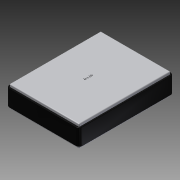
# Autodesk Inventor part: Control System_RadioRobot_DLink_DAP1522
Saved by Autodesk Inventor 2014 SP1 (Build 180222100, 222)
## iProperties
Category: Control System
Company: Autodesk Inc.
Created: 2012-12-01
Part Number: Control System_RadioRobot_DLink_DAP1522
Document SubType Name: Modeling
Designer: Autodesk Inc.
Density: 0.312319 g/cm^3
Catalog Web Link: ftp://ftp10.dlink.com/pdfs/products/DAP-1522/DAP-1522_ds.pdf
Description: Wireless bridge
Vendor: D-Link
Mass: 117.934 g
Surface Area: 482.928 cm^2
Volume: 523.554 cm^3
Material: Generic
Appearance: Glossy - Black
Author: Autodesk Inc.
Autodesk Inventor part; units mm, degrees
note: some values were not read from the file. Chosen so that the rebuilt part matches the saved one: direction of "Emboss1".
ref_plane "YZ Plane" through (0, 0, 0) normal (1, 0, 0) x (0, 1, 0)
ref_plane "XZ Plane" through (0, 0, 0) normal (0, 1, 0) x (-1, 0, 0)
ref_plane "XY Plane" through (0, 0, 0) normal (0, 0, 1) x (1, 0, 0)
sketch "Sketch1" plane through (0, 0, 0) normal (0, 0, 1) x (1, 0, 0)
  line L0 (0, 0) -> (144.78, 0)
  line L1 (144.78, 0) -> (144.78, -111.76)
  line L2 (144.78, -111.76) -> (0, -111.76)
  line L3 (0, -111.76) -> (0, 0)
  dimension "d0" = 144.78
  dimension "d1" = 111.76
  constraints: 8 end point, 2 parallel, 1 horizontal, 1 perpendicular
  measures "d0" distance of L1.end L2.end
  measures "d1" distance of L0.end L1.end
extrude "Extrusion1" add sketch "Sketch1" along normal mid plane 25.4
sketch "Sketch2" plane through (0, 0, 0) normal (0, 0, 1) x (1, 0, 0)
  line L0 (2.54, -109.22) -> (142.24, -109.22)
  line L1 (142.24, -109.22) -> (142.24, -2.54)
  line L2 (142.24, -2.54) -> (2.54, -2.54)
  line L3 (2.54, -2.54) -> (2.54, -109.22)
  line L4 (0, 0) -> (0, -111.76) projected
  line L5 (144.78, 0) -> (0, 0) projected
  dimension "d4" = 2.54
  dimension "d5" = 2.54
  dimension "d11" = 2.54
  dimension "d12" = 2.54
  constraints: 8 end point, 2 parallel, 1 horizontal, 1 perpendicular
  measures "d4" distance between parallel lines of L3 L4
  measures "d5" distance between parallel lines of L5 L2
  measures "d11" distance from line of L4.end L0
  measures "d12" distance from line of L5.start L1
extrude "Extrusion2" add sketch "Sketch2" along normal mid plane 33.02
fillet "Fillet1" radius 0.508 8 edges at (0, -55.88, 12.7) (72.39, -111.76, 12.7) (144.78, -55.88, 12.7) (72.39, 0, 12.7) (0, -55.88, -12.7) (72.39, 0, -12.7) (72.39, -111.76, -12.7) (144.78, -55.88, -12.7)
fillet "Fillet2" radius 1.27 16 edges at (2.54, -55.88, 16.51) (72.39, -2.54, 16.51) (142.24, -55.88, 16.51) (72.39, -109.22, 16.51) (2.54, -109.22, 14.605) (142.24, -109.22, 14.605) (142.24, -2.54, 14.605) (2.54, -2.54, 14.605) (2.54, -55.88, -16.51) (72.39, -109.22, -16.51) (142.24, -55.88, -16.51) (72.39, -2.54, -16.51) (142.24, -2.54, -14.605) (2.54, -2.54, -14.605) (2.54, -109.22, -14.605) (142.24, -109.22, -14.605)
fillet "Fillet3" radius 5.08 12 edges at (0.1488, -0.1488, 12.5512) (0.1488, -0.1488, -12.5512) (0, 0, 0) (0.1488, -111.6112, -12.5512) (0.1488, -111.6112, 12.5512) (0, -111.76, 0) (144.6312, -111.6112, -12.5512) (144.6312, -111.6112, 12.5512) (144.78, -111.76, 0) (144.6312, -0.1488, -12.5512) (144.6312, -0.1488, 12.5512) (144.78, 0, 0)
sketch "Sketch3" plane through (0, 0, 16.51) normal (0, 0, 1) x (1, 0, 0)
  line L0 (65.3497, -52.5642) -> (65.3318, -52.6773)
  line L1 (66.6099, -52.5642) -> (65.3497, -52.5642)
  spline S0 degree 3 poles (67.8153, -52.9891) (67.5735, -52.7056) (67.1714, -52.5642) (66.6099, -52.5642) knots 0 0 0 0 1 1 1 1
  ellipse E0 centre (41.2685, -67.4041) end of major axis (67.9555, -53.1944) minor radius 5.823 (68.0717, -54.0812) -> (67.8153, -52.9891) ccw
  ellipse E1 centre (-43.6594, 9.5813) end of major axis (67.8598, -54.6923) minor radius 14.6191 (67.4733, -55.152) -> (68.0717, -54.0812) ccw
  spline S1 degree 3 poles (66.1223, -55.5743) (66.6925, -55.5743) (67.1412, -55.435) (67.4733, -55.152) knots 0 0 0 0 1 1 1 1
  line L2 (64.873, -55.5743) -> (66.1223, -55.5743)
  line L3 (64.8909, -55.4611) -> (64.873, -55.5743)
  spline S2 degree 3 poles (65.2131, -55.368) (65.1492, -55.4241) (65.0421, -55.4545) (64.8909, -55.4611) knots 0 0 0 0 1 1 1 1
  ellipse E2 centre (64.1895, -52.8955) end of major axis (63.2262, -50.386) minor radius 0.7127 (65.2131, -55.368) -> (65.3425, -55.0693) ccw
  line L4 (65.3425, -55.0693) -> (65.6445, -53.1627)
  spline S3 degree 3 poles (65.6237, -52.7579) (65.6728, -52.8057) (65.6797, -52.9407) (65.6445, -53.1627) knots 0 0 0 0 1 1 1 1
  spline S4 degree 3 poles (65.3318, -52.6773) (65.4766, -52.6839) (65.5747, -52.71) (65.6237, -52.7579) knots 0 0 0 0 1 1 1 1
  line L5 (68.3955, -54.3728) -> (68.3503, -54.6579)
  line L6 (69.5273, -54.3728) -> (68.3955, -54.3728)
  line L7 (69.4821, -54.6579) -> (69.5273, -54.3728)
  line L8 (68.3503, -54.6579) -> (69.4821, -54.6579)
  line L9 (69.6596, -55.4611) -> (69.6417, -55.5743)
  ellipse E3 centre (57.3747, -50.2312) end of major axis (70.0338, -55.3094) minor radius 1.3637 (69.6596, -55.4611) -> (70.0293, -55.3193) ccw
  spline S5 degree 3 poles (70.1261, -54.9757) (70.1158, -55.0406) (70.1023, -55.1074) (70.0705, -55.2204) (70.0523, -55.2729) (70.0293, -55.3193) knots 0 0 0 0 0.558026 0.558026 1 1 1 1
  line L10 (70.4132, -53.1627) -> (70.1261, -54.9757)
  spline S6 degree 3 poles (70.4099, -52.7992) (70.4261, -52.8431) (70.4315, -52.8969) (70.4326, -53.0177) (70.4241, -53.0937) (70.4132, -53.1627) knots 0 0 0 0 0.421499 0.421499 1 1 1 1
  spline S7 degree 3 poles (70.1005, -52.6773) (70.2776, -52.686) (70.3824, -52.7252) (70.4099, -52.7992) knots 0 0 0 0 1 1 1 1
  line L11 (70.1184, -52.5642) -> (70.1005, -52.6773)
  line L12 (71.3677, -52.5642) -> (70.1184, -52.5642)
  line L13 (71.3498, -52.6773) -> (71.3677, -52.5642)
  spline S8 degree 3 poles (70.9984, -52.7796) (71.0444, -52.723) (71.1606, -52.6904) (71.3498, -52.6773) knots 0 0 0 0 1 1 1 1
  spline S9 degree 3 poles (70.8833, -53.1627) (70.9151, -52.9625) (70.9525, -52.8362) (70.9984, -52.7796) knots 0 0 0 0 1 1 1 1
  line L14 (70.5786, -55.0867) -> (70.8833, -53.1627)
  spline S10 degree 3 poles (70.6211, -55.3396) (70.5689, -55.3131) (70.5562, -55.2282) (70.5786, -55.0867) knots 0 0 0 0 1 1 1 1
  ellipse E4 centre (77.9872, -54.0432) end of major axis (85.3798, -52.7746) minor radius 0.4222 (70.6211, -55.3396) -> (70.9851, -55.3784) ccw
  line L15 (71.1788, -55.3784) -> (70.9851, -55.3784)
  spline S11 degree 3 poles (71.7877, -55.2717) (71.6284, -55.3435) (71.4248, -55.3784) (71.1788, -55.3784) knots 0 0 0 0 1 1 1 1
  ellipse E5 centre (72.6832, 50.9705) end of major axis (73.757, 157.2522) minor radius 6.3937 (71.7877, -55.2717) -> (72.2664, -54.7646) ccw
  line L16 (72.3774, -54.7646) -> (72.2664, -54.7646)
  line L17 (72.0206, -55.5743) -> (72.3774, -54.7646)
  line L18 (69.6417, -55.5743) -> (72.0206, -55.5743)
  line L19 (72.4733, -55.5743) -> (73.481, -55.5743)
  line L20 (72.4871, -55.4872) -> (72.4733, -55.5743)
  spline S12 degree 3 poles (72.7487, -55.4023) (72.7005, -55.4589) (72.6133, -55.4872) (72.4871, -55.4872) knots 0 0 0 0 1 1 1 1
  spline S13 degree 3 poles (72.8627, -55.0671) (72.8519, -55.135) (72.8366, -55.2089) (72.7998, -55.3171) (72.7783, -55.3675) (72.7487, -55.4023) knots 0 0 0 0 0.60012 0.60012 1 1 1 1
  line L21 (72.8627, -55.0671) -> (73.0271, -54.0289)
  ellipse E6 centre (72.1534, -55.2391) end of major axis (72.9896, -53.7975) minor radius 0.3276 (73.0271, -54.0289) -> (73.0102, -53.8161) ccw
  spline S14 degree 3 poles (72.841, -53.7612) (72.8757, -53.7612) (72.9141, -53.7643) (72.9602, -53.7793) (72.973, -53.7849) (72.9943, -53.7988) (73.0031, -53.8067) (73.0102, -53.8161) knots 0 0 0 0 0.576408 0.576408 0.803632 0.803632 1 1 1 1
  line L22 (72.7605, -53.7612) -> (72.841, -53.7612)
  line L23 (72.7742, -53.6742) -> (72.7605, -53.7612)
  line L24 (73.507, -53.4587) -> (72.7742, -53.6742)
  line L25 (73.2523, -55.0671) -> (73.507, -53.4587)
  spline S15 degree 3 poles (73.2661, -55.4159) (73.2265, -55.3675) (73.2233, -55.25) (73.2523, -55.0671) knots 0 0 0 0 1 1 1 1
  ellipse E7 centre (77.3295, -52.9371) end of major axis (81.4031, -50.4727) minor radius 0.7662 (73.2661, -55.4159) -> (73.4948, -55.4872) ccw
  line L26 (73.481, -55.5743) -> (73.4948, -55.4872)
  spline S16 degree 3 poles (73.146, -52.7013) (73.1353, -52.7687) (73.1481, -52.8253) (73.1881, -52.8716) knots 0 0 0 0 1 1 1 1
  spline S17 degree 3 poles (73.2425, -52.5315) (73.1871, -52.5794) (73.1563, -52.636) (73.146, -52.7013) knots 0 0 0 0 1 1 1 1
  spline S18 degree 3 poles (73.4258, -52.4597) (73.3584, -52.4597) (73.298, -52.4836) (73.2425, -52.5315) knots 0 0 0 0 1 1 1 1
  spline S19 degree 3 poles (73.5821, -52.5315) (73.5418, -52.4836) (73.4911, -52.4597) (73.4258, -52.4597) knots 0 0 0 0 1 1 1 1
  spline S20 degree 3 poles (73.627, -52.7013) (73.6373, -52.636) (73.6224, -52.5794) (73.5821, -52.5315) knots 0 0 0 0 1 1 1 1
  ellipse E8 centre (71.9698, -51.7105) end of major axis (73.582, -52.8173) minor radius 0.7104 (73.5276, -52.8754) -> (73.627, -52.7013) ccw
  spline S21 degree 3 poles (73.3497, -52.9407) (73.415, -52.9407) (73.4728, -52.9189) (73.5276, -52.8754) knots 0 0 0 0 1 1 1 1
  spline S22 degree 3 poles (73.1881, -52.8716) (73.229, -52.9189) (73.2822, -52.9407) (73.3497, -52.9407) knots 0 0 0 0 1 1 1 1
  line L27 (73.6167, -55.4872) -> (73.6029, -55.5743)
  spline S23 degree 3 poles (73.8749, -55.3852) (73.8199, -55.4545) (73.7342, -55.4872) (73.6167, -55.4872) knots 0 0 0 0 1 1 1 1
  spline S24 degree 3 poles (73.9923, -55.0671) (73.9824, -55.1294) (73.9678, -55.1936) (73.9288, -55.2992) (73.9058, -55.3464) (73.8749, -55.3852) knots 0 0 0 0 0.558687 0.558687 1 1 1 1
  line L28 (73.9923, -55.0671) -> (74.1609, -54.0028)
  spline S25 degree 3 poles (74.1506, -53.82) (74.1706, -53.8592) (74.174, -53.9201) (74.1609, -54.0028) knots 0 0 0 0 1 1 1 1
  spline S26 degree 3 poles (74.0163, -53.7612) (74.0859, -53.7612) (74.1307, -53.7808) (74.1506, -53.82) knots 0 0 0 0 1 1 1 1
  line L29 (73.8901, -53.7612) -> (74.0163, -53.7612)
  line L30 (73.9038, -53.6742) -> (73.8901, -53.7612)
  line L31 (74.6366, -53.4587) -> (73.9038, -53.6742)
  line L32 (74.5839, -53.7917) -> (74.6366, -53.4587)
  spline S27 degree 3 poles (74.9832, -53.524) (74.8806, -53.5675) (74.7489, -53.6568) (74.5839, -53.7917) knots 0 0 0 0 1 1 1 1
  spline S28 degree 3 poles (75.2918, -53.4587) (75.1873, -53.4587) (75.0859, -53.4805) (74.9832, -53.524) knots 0 0 0 0 1 1 1 1
  ellipse E9 centre (69.491, -60.1714) end of major axis (63.3694, -66.779) minor radius 1.7408 (75.6688, -53.6311) -> (75.2918, -53.4587) ccw
  ellipse E10 centre (64.3467, -63.1911) end of major axis (75.6367, -53.5878) minor radius 2.4275 (75.7313, -54.1051) -> (75.6688, -53.6311) ccw
  line L33 (75.7313, -54.1051) -> (75.579, -55.0671)
  ellipse E11 centre (79.0817, -48.7921) end of major axis (82.5408, -42.1531) minor radius 0.7356 (75.579, -55.0671) -> (75.6022, -55.4154) ccw
  spline S29 degree 3 poles (75.8215, -55.4872) (75.7192, -55.4872) (75.6468, -55.4633) (75.6022, -55.4154) knots 0 0 0 0 1 1 1 1
  line L34 (75.8077, -55.5743) -> (75.8215, -55.4872)
  line L35 (74.8, -55.5743) -> (75.8077, -55.5743)
  line L36 (74.8138, -55.4872) -> (74.8, -55.5743)
  spline S30 degree 3 poles (75.0576, -55.4148) (74.9982, -55.4633) (74.9182, -55.4872) (74.8138, -55.4872) knots 0 0 0 0 1 1 1 1
  ellipse E12 centre (74.402, -53.5777) end of major axis (73.7975, -51.7123) minor radius 0.5398 (75.0576, -55.4148) -> (75.178, -55.139) ccw
  line L37 (75.178, -55.139) -> (75.3266, -54.2009)
  ellipse E13 centre (55.6406, -76.8384) end of major axis (75.2465, -53.7648) minor radius 2.5286 (75.3266, -54.2009) -> (75.0609, -53.7068) ccw
  ellipse E14 centre (70.9828, -106.1576) end of major axis (75.0958, -53.7082) minor radius 4.8337 (75.0609, -53.7068) -> (74.6474, -53.8853) ccw
  line L38 (74.5573, -53.9593) -> (74.6474, -53.8853)
  line L39 (74.3819, -55.0671) -> (74.5573, -53.9593)
  spline S31 degree 3 poles (74.4075, -55.4001) (74.3639, -55.3457) (74.3553, -55.2347) (74.3819, -55.0671) knots 0 0 0 0 1 1 1 1
  ellipse E15 centre (77.9499, -52.5696) end of major axis (81.4925, -49.7392) minor radius 0.9098 (74.4075, -55.4001) -> (74.6244, -55.4872) ccw
  line L40 (74.6106, -55.5743) -> (74.6244, -55.4872)
  line L41 (73.6029, -55.5743) -> (74.6106, -55.5743)
  line L42 (75.8607, -55.4872) -> (75.8469, -55.5743)
  spline S32 degree 3 poles (76.1147, -55.4088) (76.0636, -55.4567) (75.9789, -55.4828) (75.8607, -55.4872) knots 0 0 0 0 1 1 1 1
  spline S33 degree 3 poles (76.2194, -55.1738) (76.2119, -55.2209) (76.1998, -55.2692) (76.1644, -55.3485) (76.1432, -55.3822) (76.1147, -55.4088) knots 0 0 0 0 0.549628 0.549628 1 1 1 1
  line L43 (76.2194, -55.1738) -> (76.5386, -53.1583)
  spline S34 degree 3 poles (76.5308, -52.8776) (76.5577, -52.9276) (76.5603, -53.0212) (76.5386, -53.1583) knots 0 0 0 0 1 1 1 1
  spline S35 degree 3 poles (76.384, -52.8014) (76.4558, -52.8014) (76.5039, -52.8275) (76.5308, -52.8776) knots 0 0 0 0 1 1 1 1
  spline S36 degree 3 poles (76.2857, -52.8036) (76.3184, -52.8036) (76.3514, -52.8014) (76.384, -52.8014) knots 0 0 0 0 1 1 1 1
  line L44 (76.2995, -52.7165) -> (76.2857, -52.8036)
  line L45 (77.0323, -52.501) -> (76.2995, -52.7165)
  line L46 (76.7379, -54.3598) -> (77.0323, -52.501)
  line L47 (77.2838, -53.9223) -> (76.7379, -54.3598)
  spline S37 degree 3 poles (77.4969, -53.7411) (77.4715, -53.7678) (77.4008, -53.8285) (77.2838, -53.9223) knots 0 0 0 0 1 1 1 1
  spline S38 degree 3 poles (77.54, -53.6655) (77.5358, -53.6916) (77.5212, -53.7155) (77.4969, -53.7411) knots 0 0 0 0 1 1 1 1
  spline S39 degree 3 poles (77.5186, -53.6183) (77.5346, -53.6306) (77.5431, -53.6459) (77.54, -53.6655) knots 0 0 0 0 1 1 1 1
  spline S40 degree 3 poles (77.3344, -53.5893) (77.4418, -53.598) (77.5036, -53.6067) (77.5186, -53.6183) knots 0 0 0 0 1 1 1 1
  line L48 (77.3482, -53.5022) -> (77.3344, -53.5893)
  line L49 (78.2776, -53.5022) -> (77.3482, -53.5022)
  line L50 (78.2638, -53.5893) -> (78.2776, -53.5022)
  spline S41 degree 3 poles (77.8006, -53.7242) (77.9221, -53.6437) (78.0752, -53.598) (78.2638, -53.5893) knots 0 0 0 0 1 1 1 1
  spline S42 degree 3 poles (77.4886, -53.9484) (77.5737, -53.8788) (77.679, -53.8048) (77.8006, -53.7242) knots 0 0 0 0 1 1 1 1
  line L51 (77.0662, -54.2792) -> (77.4886, -53.9484)
  line L52 (77.4682, -54.9844) -> (77.0662, -54.2792)
  spline S43 degree 3 poles (77.7521, -55.3745) (77.6685, -55.3) (77.5745, -55.1709) (77.4682, -54.9844) knots 0 0 0 0 1 1 1 1
  ellipse E16 centre (83.8098, -40.0957) end of major axis (89.7321, -24.7331) minor radius 2.6176 (77.7521, -55.3745) -> (78.048, -55.4872) ccw
  line L53 (78.0343, -55.5743) -> (78.048, -55.4872)
  line L54 (77.0548, -55.5743) -> (78.0343, -55.5743)
  line L55 (77.0686, -55.4872) -> (77.0548, -55.5743)
  spline S44 degree 3 poles (77.2031, -55.476) (77.1756, -55.485) (77.1317, -55.4872) (77.0686, -55.4872) knots 0 0 0 0 1 1 1 1
  spline S45 degree 3 poles (77.2467, -55.435) (77.2436, -55.4545) (77.2284, -55.4676) (77.2031, -55.476) knots 0 0 0 0 1 1 1 1
  spline S46 degree 3 poles (77.2216, -55.3549) (77.2313, -55.3721) (77.2381, -55.3876) (77.2442, -55.407) (77.2458, -55.4135) (77.2472, -55.4247) (77.2474, -55.43) (77.2467, -55.435) knots 0 0 0 0 0.552394 0.552394 0.803155 0.803155 1 1 1 1
  spline S47 degree 3 poles (77.1348, -55.1934) (77.1731, -55.2674) (77.2018, -55.3196) (77.2216, -55.3549) knots 0 0 0 0 1 1 1 1
  line L56 (76.7238, -54.449) -> (77.1348, -55.1934)
  line L57 (76.6259, -55.0671) -> (76.7238, -54.449)
  spline S48 degree 3 poles (76.6204, -55.4097) (76.5942, -55.3631) (76.5969, -55.25) (76.6259, -55.0671) knots 0 0 0 0 1 1 1 1
  ellipse E17 centre (82.6616, -53.1831) end of major axis (88.7076, -50.967) minor radius 0.6738 (76.6204, -55.4097) -> (76.8684, -55.4872) ccw
  line L58 (76.8546, -55.5743) -> (76.8684, -55.4872)
  line L59 (75.8469, -55.5743) -> (76.8546, -55.5743)
  spline S49 degree 3 poles (66.4548, -52.76) (66.8771, -52.76) (67.1767, -52.8885) (67.3587, -53.1409) knots 0 0 0 0 1 1 1 1
  line L60 (65.3497, -52.5642) -> (65.3318, -52.6773)
  line L61 (66.6099, -52.5642) -> (65.3497, -52.5642)
  spline S50 degree 3 poles (67.8153, -52.9891) (67.5735, -52.7056) (67.1714, -52.5642) (66.6099, -52.5642) knots 0 0 0 0 1 1 1 1
  ellipse E18 centre (41.2685, -67.4041) end of major axis (67.9555, -53.1944) minor radius 5.823 (68.0717, -54.0812) -> (67.8153, -52.9891) ccw
  ellipse E19 centre (-43.6594, 9.5813) end of major axis (67.8598, -54.6923) minor radius 14.6191 (67.4733, -55.152) -> (68.0717, -54.0812) ccw
  spline S51 degree 3 poles (66.1223, -55.5743) (66.6925, -55.5743) (67.1412, -55.435) (67.4733, -55.152) knots 0 0 0 0 1 1 1 1
  line L62 (64.873, -55.5743) -> (66.1223, -55.5743)
  line L63 (64.8909, -55.4611) -> (64.873, -55.5743)
  spline S52 degree 3 poles (65.2131, -55.368) (65.1492, -55.4241) (65.0421, -55.4545) (64.8909, -55.4611) knots 0 0 0 0 1 1 1 1
  ellipse E20 centre (64.1895, -52.8955) end of major axis (63.2262, -50.386) minor radius 0.7127 (65.2131, -55.368) -> (65.3425, -55.0693) ccw
  line L64 (65.3425, -55.0693) -> (65.6445, -53.1627)
  spline S53 degree 3 poles (65.6237, -52.7579) (65.6728, -52.8057) (65.6797, -52.9407) (65.6445, -53.1627) knots 0 0 0 0 1 1 1 1
  spline S54 degree 3 poles (65.3318, -52.6773) (65.4766, -52.6839) (65.5747, -52.71) (65.6237, -52.7579) knots 0 0 0 0 1 1 1 1
  line L65 (68.3955, -54.3728) -> (68.3503, -54.6579)
  line L66 (69.5273, -54.3728) -> (68.3955, -54.3728)
  line L67 (69.4821, -54.6579) -> (69.5273, -54.3728)
  line L68 (68.3503, -54.6579) -> (69.4821, -54.6579)
  line L69 (69.6596, -55.4611) -> (69.6417, -55.5743)
  ellipse E21 centre (57.3747, -50.2312) end of major axis (70.0338, -55.3094) minor radius 1.3637 (69.6596, -55.4611) -> (70.0293, -55.3193) ccw
  spline S55 degree 3 poles (70.1261, -54.9757) (70.1158, -55.0406) (70.1023, -55.1074) (70.0705, -55.2204) (70.0523, -55.2729) (70.0293, -55.3193) knots 0 0 0 0 0.558026 0.558026 1 1 1 1
  line L70 (70.4132, -53.1627) -> (70.1261, -54.9757)
  spline S56 degree 3 poles (70.4099, -52.7992) (70.4261, -52.8431) (70.4315, -52.8969) (70.4326, -53.0177) (70.4241, -53.0937) (70.4132, -53.1627) knots 0 0 0 0 0.421499 0.421499 1 1 1 1
  spline S57 degree 3 poles (70.1005, -52.6773) (70.2776, -52.686) (70.3824, -52.7252) (70.4099, -52.7992) knots 0 0 0 0 1 1 1 1
  line L71 (70.1184, -52.5642) -> (70.1005, -52.6773)
  line L72 (71.3677, -52.5642) -> (70.1184, -52.5642)
  line L73 (71.3498, -52.6773) -> (71.3677, -52.5642)
  spline S58 degree 3 poles (70.9984, -52.7796) (71.0444, -52.723) (71.1606, -52.6904) (71.3498, -52.6773) knots 0 0 0 0 1 1 1 1
  spline S59 degree 3 poles (70.8833, -53.1627) (70.9151, -52.9625) (70.9525, -52.8362) (70.9984, -52.7796) knots 0 0 0 0 1 1 1 1
  line L74 (70.5786, -55.0867) -> (70.8833, -53.1627)
  spline S60 degree 3 poles (70.6211, -55.3396) (70.5689, -55.3131) (70.5562, -55.2282) (70.5786, -55.0867) knots 0 0 0 0 1 1 1 1
  ellipse E22 centre (77.9872, -54.0432) end of major axis (85.3798, -52.7746) minor radius 0.4222 (70.6211, -55.3396) -> (70.9851, -55.3784) ccw
  line L75 (71.1788, -55.3784) -> (70.9851, -55.3784)
  spline S61 degree 3 poles (71.7877, -55.2717) (71.6284, -55.3435) (71.4248, -55.3784) (71.1788, -55.3784) knots 0 0 0 0 1 1 1 1
  ellipse E23 centre (72.6832, 50.9705) end of major axis (73.757, 157.2522) minor radius 6.3937 (71.7877, -55.2717) -> (72.2664, -54.7646) ccw
  line L76 (72.3774, -54.7646) -> (72.2664, -54.7646)
  line L77 (72.0206, -55.5743) -> (72.3774, -54.7646)
  line L78 (69.6417, -55.5743) -> (72.0206, -55.5743)
  line L79 (72.4733, -55.5743) -> (73.481, -55.5743)
  line L80 (72.4871, -55.4872) -> (72.4733, -55.5743)
  spline S62 degree 3 poles (72.7487, -55.4023) (72.7005, -55.4589) (72.6133, -55.4872) (72.4871, -55.4872) knots 0 0 0 0 1 1 1 1
  spline S63 degree 3 poles (72.8627, -55.0671) (72.8519, -55.135) (72.8366, -55.2089) (72.7998, -55.3171) (72.7783, -55.3675) (72.7487, -55.4023) knots 0 0 0 0 0.60012 0.60012 1 1 1 1
  line L81 (72.8627, -55.0671) -> (73.0271, -54.0289)
  ellipse E24 centre (72.1534, -55.2391) end of major axis (72.9896, -53.7975) minor radius 0.3276 (73.0271, -54.0289) -> (73.0102, -53.8161) ccw
  spline S64 degree 3 poles (72.841, -53.7612) (72.8757, -53.7612) (72.9141, -53.7643) (72.9602, -53.7793) (72.973, -53.7849) (72.9943, -53.7988) (73.0031, -53.8067) (73.0102, -53.8161) knots 0 0 0 0 0.576408 0.576408 0.803632 0.803632 1 1 1 1
  line L82 (72.7605, -53.7612) -> (72.841, -53.7612)
  line L83 (72.7742, -53.6742) -> (72.7605, -53.7612)
  line L84 (73.507, -53.4587) -> (72.7742, -53.6742)
  line L85 (73.2523, -55.0671) -> (73.507, -53.4587)
  spline S65 degree 3 poles (73.2661, -55.4159) (73.2265, -55.3675) (73.2233, -55.25) (73.2523, -55.0671) knots 0 0 0 0 1 1 1 1
  ellipse E25 centre (77.3295, -52.9371) end of major axis (81.4031, -50.4727) minor radius 0.7662 (73.2661, -55.4159) -> (73.4948, -55.4872) ccw
  line L86 (73.481, -55.5743) -> (73.4948, -55.4872)
  spline S66 degree 3 poles (73.146, -52.7013) (73.1353, -52.7687) (73.1481, -52.8253) (73.1881, -52.8716) knots 0 0 0 0 1 1 1 1
  spline S67 degree 3 poles (73.2425, -52.5315) (73.1871, -52.5794) (73.1563, -52.636) (73.146, -52.7013) knots 0 0 0 0 1 1 1 1
  spline S68 degree 3 poles (73.4258, -52.4597) (73.3584, -52.4597) (73.298, -52.4836) (73.2425, -52.5315) knots 0 0 0 0 1 1 1 1
  spline S69 degree 3 poles (73.5821, -52.5315) (73.5418, -52.4836) (73.4911, -52.4597) (73.4258, -52.4597) knots 0 0 0 0 1 1 1 1
  spline S70 degree 3 poles (73.627, -52.7013) (73.6373, -52.636) (73.6224, -52.5794) (73.5821, -52.5315) knots 0 0 0 0 1 1 1 1
  ellipse E26 centre (71.9698, -51.7105) end of major axis (73.582, -52.8173) minor radius 0.7104 (73.5276, -52.8754) -> (73.627, -52.7013) ccw
  spline S71 degree 3 poles (73.3497, -52.9407) (73.415, -52.9407) (73.4728, -52.9189) (73.5276, -52.8754) knots 0 0 0 0 1 1 1 1
  spline S72 degree 3 poles (73.1881, -52.8716) (73.229, -52.9189) (73.2822, -52.9407) (73.3497, -52.9407) knots 0 0 0 0 1 1 1 1
  line L87 (73.6167, -55.4872) -> (73.6029, -55.5743)
  spline S73 degree 3 poles (73.8749, -55.3852) (73.8199, -55.4545) (73.7342, -55.4872) (73.6167, -55.4872) knots 0 0 0 0 1 1 1 1
  spline S74 degree 3 poles (73.9923, -55.0671) (73.9824, -55.1294) (73.9678, -55.1936) (73.9288, -55.2992) (73.9058, -55.3464) (73.8749, -55.3852) knots 0 0 0 0 0.558687 0.558687 1 1 1 1
  line L88 (73.9923, -55.0671) -> (74.1609, -54.0028)
  spline S75 degree 3 poles (74.1506, -53.82) (74.1706, -53.8592) (74.174, -53.9201) (74.1609, -54.0028) knots 0 0 0 0 1 1 1 1
  spline S76 degree 3 poles (74.0163, -53.7612) (74.0859, -53.7612) (74.1307, -53.7808) (74.1506, -53.82) knots 0 0 0 0 1 1 1 1
  line L89 (73.8901, -53.7612) -> (74.0163, -53.7612)
  line L90 (73.9038, -53.6742) -> (73.8901, -53.7612)
  line L91 (74.6366, -53.4587) -> (73.9038, -53.6742)
  line L92 (74.5839, -53.7917) -> (74.6366, -53.4587)
  spline S77 degree 3 poles (74.9832, -53.524) (74.8806, -53.5675) (74.7489, -53.6568) (74.5839, -53.7917) knots 0 0 0 0 1 1 1 1
  spline S78 degree 3 poles (75.2918, -53.4587) (75.1873, -53.4587) (75.0859, -53.4805) (74.9832, -53.524) knots 0 0 0 0 1 1 1 1
  ellipse E27 centre (69.491, -60.1714) end of major axis (63.3694, -66.779) minor radius 1.7408 (75.6688, -53.6311) -> (75.2918, -53.4587) ccw
  ellipse E28 centre (64.3467, -63.1911) end of major axis (75.6367, -53.5878) minor radius 2.4275 (75.7313, -54.1051) -> (75.6688, -53.6311) ccw
  line L93 (75.7313, -54.1051) -> (75.579, -55.0671)
  ellipse E29 centre (79.0817, -48.7921) end of major axis (82.5408, -42.1531) minor radius 0.7356 (75.579, -55.0671) -> (75.6022, -55.4154) ccw
  spline S79 degree 3 poles (75.8215, -55.4872) (75.7192, -55.4872) (75.6468, -55.4633) (75.6022, -55.4154) knots 0 0 0 0 1 1 1 1
  line L94 (75.8077, -55.5743) -> (75.8215, -55.4872)
  line L95 (74.8, -55.5743) -> (75.8077, -55.5743)
  line L96 (74.8138, -55.4872) -> (74.8, -55.5743)
  spline S80 degree 3 poles (75.0576, -55.4148) (74.9982, -55.4633) (74.9182, -55.4872) (74.8138, -55.4872) knots 0 0 0 0 1 1 1 1
  ellipse E30 centre (74.402, -53.5777) end of major axis (73.7975, -51.7123) minor radius 0.5398 (75.0576, -55.4148) -> (75.178, -55.139) ccw
  line L97 (75.178, -55.139) -> (75.3266, -54.2009)
  ellipse E31 centre (55.6406, -76.8384) end of major axis (75.2465, -53.7648) minor radius 2.5286 (75.3266, -54.2009) -> (75.0609, -53.7068) ccw
  ellipse E32 centre (70.9828, -106.1576) end of major axis (75.0958, -53.7082) minor radius 4.8337 (75.0609, -53.7068) -> (74.6474, -53.8853) ccw
  line L98 (74.5573, -53.9593) -> (74.6474, -53.8853)
  line L99 (74.3819, -55.0671) -> (74.5573, -53.9593)
  spline S81 degree 3 poles (74.4075, -55.4001) (74.3639, -55.3457) (74.3553, -55.2347) (74.3819, -55.0671) knots 0 0 0 0 1 1 1 1
  ellipse E33 centre (77.9499, -52.5696) end of major axis (81.4925, -49.7392) minor radius 0.9098 (74.4075, -55.4001) -> (74.6244, -55.4872) ccw
  line L100 (74.6106, -55.5743) -> (74.6244, -55.4872)
  line L101 (73.6029, -55.5743) -> (74.6106, -55.5743)
  line L102 (75.8607, -55.4872) -> (75.8469, -55.5743)
  spline S82 degree 3 poles (76.1147, -55.4088) (76.0636, -55.4567) (75.9789, -55.4828) (75.8607, -55.4872) knots 0 0 0 0 1 1 1 1
  spline S83 degree 3 poles (76.2194, -55.1738) (76.2119, -55.2209) (76.1998, -55.2692) (76.1644, -55.3485) (76.1432, -55.3822) (76.1147, -55.4088) knots 0 0 0 0 0.549628 0.549628 1 1 1 1
  line L103 (76.2194, -55.1738) -> (76.5386, -53.1583)
  spline S84 degree 3 poles (76.5308, -52.8776) (76.5577, -52.9276) (76.5603, -53.0212) (76.5386, -53.1583) knots 0 0 0 0 1 1 1 1
  spline S85 degree 3 poles (76.384, -52.8014) (76.4558, -52.8014) (76.5039, -52.8275) (76.5308, -52.8776) knots 0 0 0 0 1 1 1 1
  spline S86 degree 3 poles (76.2857, -52.8036) (76.3184, -52.8036) (76.3514, -52.8014) (76.384, -52.8014) knots 0 0 0 0 1 1 1 1
  line L104 (76.2995, -52.7165) -> (76.2857, -52.8036)
  line L105 (77.0323, -52.501) -> (76.2995, -52.7165)
  line L106 (76.7379, -54.3598) -> (77.0323, -52.501)
  line L107 (77.2838, -53.9223) -> (76.7379, -54.3598)
  spline S87 degree 3 poles (77.4969, -53.7411) (77.4715, -53.7678) (77.4008, -53.8285) (77.2838, -53.9223) knots 0 0 0 0 1 1 1 1
  spline S88 degree 3 poles (77.54, -53.6655) (77.5358, -53.6916) (77.5212, -53.7155) (77.4969, -53.7411) knots 0 0 0 0 1 1 1 1
  spline S89 degree 3 poles (77.5186, -53.6183) (77.5346, -53.6306) (77.5431, -53.6459) (77.54, -53.6655) knots 0 0 0 0 1 1 1 1
  spline S90 degree 3 poles (77.3344, -53.5893) (77.4418, -53.598) (77.5036, -53.6067) (77.5186, -53.6183) knots 0 0 0 0 1 1 1 1
  line L108 (77.3482, -53.5022) -> (77.3344, -53.5893)
  line L109 (78.2776, -53.5022) -> (77.3482, -53.5022)
  line L110 (78.2638, -53.5893) -> (78.2776, -53.5022)
  spline S91 degree 3 poles (77.8006, -53.7242) (77.9221, -53.6437) (78.0752, -53.598) (78.2638, -53.5893) knots 0 0 0 0 1 1 1 1
  spline S92 degree 3 poles (77.4886, -53.9484) (77.5737, -53.8788) (77.679, -53.8048) (77.8006, -53.7242) knots 0 0 0 0 1 1 1 1
  line L111 (77.0662, -54.2792) -> (77.4886, -53.9484)
  line L112 (77.4682, -54.9844) -> (77.0662, -54.2792)
  spline S93 degree 3 poles (77.7521, -55.3745) (77.6685, -55.3) (77.5745, -55.1709) (77.4682, -54.9844) knots 0 0 0 0 1 1 1 1
  ellipse E34 centre (83.8098, -40.0957) end of major axis (89.7321, -24.7331) minor radius 2.6176 (77.7521, -55.3745) -> (78.048, -55.4872) ccw
  line L113 (78.0343, -55.5743) -> (78.048, -55.4872)
  line L114 (77.0548, -55.5743) -> (78.0343, -55.5743)
  line L115 (77.0686, -55.4872) -> (77.0548, -55.5743)
  spline S94 degree 3 poles (77.2031, -55.476) (77.1756, -55.485) (77.1317, -55.4872) (77.0686, -55.4872) knots 0 0 0 0 1 1 1 1
  spline S95 degree 3 poles (77.2467, -55.435) (77.2436, -55.4545) (77.2284, -55.4676) (77.2031, -55.476) knots 0 0 0 0 1 1 1 1
  spline S96 degree 3 poles (77.2216, -55.3549) (77.2313, -55.3721) (77.2381, -55.3876) (77.2442, -55.407) (77.2458, -55.4135) (77.2472, -55.4247) (77.2474, -55.43) (77.2467, -55.435) knots 0 0 0 0 0.552394 0.552394 0.803155 0.803155 1 1 1 1
  spline S97 degree 3 poles (77.1348, -55.1934) (77.1731, -55.2674) (77.2018, -55.3196) (77.2216, -55.3549) knots 0 0 0 0 1 1 1 1
  line L116 (76.7238, -54.449) -> (77.1348, -55.1934)
  line L117 (76.6259, -55.0671) -> (76.7238, -54.449)
  spline S98 degree 3 poles (76.6204, -55.4097) (76.5942, -55.3631) (76.5969, -55.25) (76.6259, -55.0671) knots 0 0 0 0 1 1 1 1
  ellipse E35 centre (82.6616, -53.1831) end of major axis (88.7076, -50.967) minor radius 0.6738 (76.6204, -55.4097) -> (76.8684, -55.4872) ccw
  line L118 (76.8546, -55.5743) -> (76.8684, -55.4872)
  line L119 (75.8469, -55.5743) -> (76.8546, -55.5743)
  spline S99 degree 3 poles (67.3587, -53.1409) (67.5407, -53.3934) (67.601, -53.7133) (67.5397, -54.1008) knots 0 0 0 0 1 1 1 1
  spline S100 degree 3 poles (67.5397, -54.1008) (67.4804, -54.4751) (67.3255, -54.7798) (67.0764, -55.0192) knots 0 0 0 0 1 1 1 1
  spline S101 degree 3 poles (67.0764, -55.0192) (66.8274, -55.2587) (66.4537, -55.3784) (65.9552, -55.3784) knots 0 0 0 0 1 1 1 1
  spline S102 degree 3 poles (65.9552, -55.3784) (65.8725, -55.3784) (65.8198, -55.3675) (65.8013, -55.3441) knots 0 0 0 0 1 1 1 1
  ellipse E36 centre (66.5663, -54.0542) end of major axis (67.3198, -52.7542) minor radius 0.2406 (65.7906, -55.2086) -> (65.8013, -55.3441) ccw
  line L120 (66.147, -52.9581) -> (65.7906, -55.2086)
  line L121 (66.147, -52.9581) -> (65.7906, -55.2086)
  ellipse E37 centre (66.5663, -54.0542) end of major axis (67.3198, -52.7542) minor radius 0.2406 (65.7906, -55.2086) -> (65.8013, -55.3441) ccw
  spline S103 degree 3 poles (65.9552, -55.3784) (65.8725, -55.3784) (65.8198, -55.3675) (65.8013, -55.3441) knots 0 0 0 0 1 1 1 1
  spline S104 degree 3 poles (67.0764, -55.0192) (66.8274, -55.2587) (66.4537, -55.3784) (65.9552, -55.3784) knots 0 0 0 0 1 1 1 1
  spline S105 degree 3 poles (67.5397, -54.1008) (67.4804, -54.4751) (67.3255, -54.7798) (67.0764, -55.0192) knots 0 0 0 0 1 1 1 1
  spline S106 degree 3 poles (67.3587, -53.1409) (67.5407, -53.3934) (67.601, -53.7133) (67.5397, -54.1008) knots 0 0 0 0 1 1 1 1
  spline S107 degree 3 poles (66.4548, -52.76) (66.8771, -52.76) (67.1767, -52.8885) (67.3587, -53.1409) knots 0 0 0 0 1 1 1 1
  ellipse E38 centre (69.1331, -53.6028) end of major axis (72.0663, -54.3816) minor radius 0.333 (66.4548, -52.76) -> (66.2179, -52.7992) ccw
  spline S108 degree 3 poles (66.147, -52.9581) (66.1598, -52.8776) (66.1833, -52.8253) (66.2179, -52.7992) knots 0 0 0 0 1 1 1 1
  point P0 (0, 0)
  point P1 (71.5753, -54.0453)
  point P2 (66.6074, -52.766)
  point P3 (67.3914, -53.1891)
  point P4 (67.1654, -54.9264)
  point P5 (66.6094, -55.2886)
  point P6 (65.8751, -55.3737)
  constraints: 244 end point, 493 other
emboss "Emboss1" sketch "Sketch3" operation cut depth 2.54 direction (0, 0, -1)
equation "\"d11\" = d5"
equation "\"d12\" = d5"
body "Solid2"
